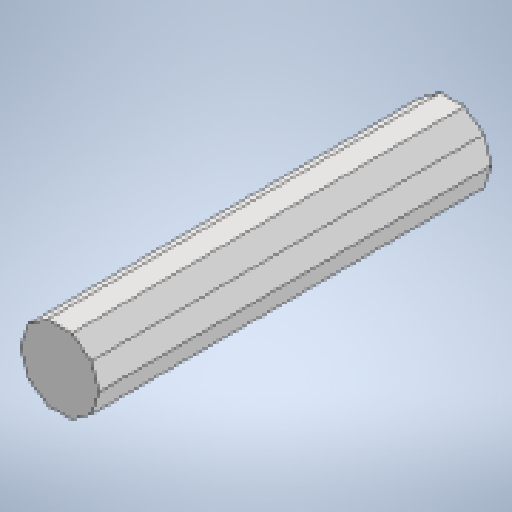
# Autodesk Inventor part: plate_joint_shaft
Saved by Autodesk Inventor 2026.2 (Build 302298000, 298)
## iProperties
Created: 2026-01-26
Part Number: plate_joint_shaft
Material: Generic
Document SubType Name: Modeling
Designer: gakut
Density: 1 g/cm^3
Appearance: Default
Author: gakut
Autodesk Inventor part; units mm, degrees
ref_plane "YZ Plane" through (0, 0, 0) normal (1, 0, 0) x (0, 1, 0)
ref_plane "XZ Plane" through (0, 0, 0) normal (0, 1, 0) x (-1, 0, 0)
ref_plane "XY Plane" through (0, 0, 0) normal (0, 0, 1) x (1, 0, 0)
sketch "Sketch1" plane through (0, 0, 0) normal (0, 0, 1) x (1, 0, 0)
  circle A0 centre (0, 0) radius 4
  line L0 (-2.6458, -3) -> (2.6458, -3)
  dimension "d3" = 8
  dimension "d4" = 1
  constraints: 2 coincident, 2 end point, 2 point on circle, 1 centre point, 1 horizontal
  measures "d3" diameter of A0
  measures "d4" distance edge to line of A0 L0
extrude "Extrusion1" add sketch "Sketch1" along normal blind 30 contours A0 L0 picked at (1.0912, -0.393)
body "Solid1"
